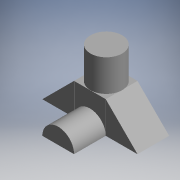
# Autodesk Inventor part: orthographic1
Saved by Autodesk Inventor 2017 (Build 210142000, 142)
## iProperties
Part Number: orthographic1
Material: Generic
Document SubType Name: Modeling
Designer: qthuynh
Appearance: Generic
Author: qthuynh
Autodesk Inventor part; units mm, degrees
ref_plane "YZ Plane" through (0, 0, 0) normal (1, 0, 0) x (0, 1, 0)
ref_plane "XZ Plane" through (0, 0, 0) normal (0, 1, 0) x (-1, 0, 0)
sketch "Sketch1" plane through (0, 0, 0) normal (0, 0, 1) x (1, 0, 0)
  line L0 (0, 0) -> (25.4, 0)
  line L1 (25.4, 0) -> (25.4, 25.4)
  line L2 (25.4, 25.4) -> (0, 25.4)
  line L3 (0, 25.4) -> (0, 0)
  line L4 (25.4, 0) -> (50.8, 0)
  line L5 (50.8, 0) -> (25.4, 25.4)
  line L6 (0, 0) -> (-25.4, 0)
  line L7 (-25.4, 0) -> (0, 25.4)
  dimension "d0" = 25.4
  dimension "d1" = 25.4
  dimension "d2" = 25.4
  dimension "d3" = 25.4
  constraints: 16 end point, 2 horizontal, 2 parallel, 2 perpendicular, 2 point on line
  measures "d0" distance of L2.end L1.end
  measures "d1" distance of L1.end L0.end
  measures "d2" distance of L0.end L4.end
  measures "d3" distance of L0.start L6.end
extrude "Extrusion1" add sketch "Sketch1" along normal blind 25.4 contours L3 L2 L1 L0
chamfer "Chamfer1" distance 0.3 angle 45 2 edges at (25.4, 12.7, 25.4) (0, 12.7, 25.4)
sketch "Sketch2" plane through (0, 0, 25.4) normal (0, 0, 1) x (1, 0, 0)
  line L0 (0, 0) -> (-25.4, 0)
  line L1 (0, 25.4) -> (0, 0) projected
  line L2 (-25.4, 0) -> (0, 25.4)
  line L3 (25.4, 0) -> (50.8, 0)
  line L4 (50.8, 0) -> (25.4, 25.4)
  dimension "d9" = 25.4
  dimension "d10" = 25.4
  constraints: 8 end point, 2 horizontal
  measures "d9" distance of L0.start L0.end
  measures "d10" distance of L3.start L3.end
extrude "Extrusion2" add sketch "Sketch2" against normal blind 25.4
sketch "Sketch3" plane through (0, 0, 25.4) normal (0, 0, 1) x (1, 0, 0)
  line L0 (-25.4, 0) -> (25.4, 0) projected
  line L1 (25.4, 0) -> (50.8, 0)
  line L2 (25.4, 0) -> (25.4, 25.4) projected
  line L3 (50.8, 0) -> (25.4, 25.4)
  point P0 (0, 0)
  dimension "d13" = 25.4
  constraints: 4 end point, 1 horizontal
  measures "d13" distance of L0.end L1.end
extrude "Extrusion3" add sketch "Sketch3" against normal blind 25.4
sketch "Sketch4" plane through (0, 0, 25.4) normal (0, 0, 1) x (1, 0, 0)
  line L0 (0.3, 0) -> (25.1, 0) projected
  circle A0 centre (12.7, 0) radius 12.7
  point P0 (0, 0)
  dimension "d16" = 25.4
  constraints: 1 centre point, 1 midpoint
  measures "d16" diameter of A0
extrude "Extrusion4" add sketch "Sketch4" along normal blind 25.4
ref_plane "Work Plane1" through (0, 0, 25.4) normal (0, 0, 1) x (1, 0, 0)
sketch "Sketch5" plane through (0, 0, 25.4) normal (0, 0, 1) x (1, 0, 0)
  line L0 (0, 0) -> (-25.4, 0) projected
  line L1 (0, 0) -> (42.4435, 0)
  line L2 (42.4435, 0) -> (42.4435, -16.3705)
  line L3 (42.4435, -16.3705) -> (0, -16.3705)
  line L4 (0, -16.3705) -> (0, 0)
  circle A0 centre (12.7, 0) radius 12.7 projected
  constraints: 8 end point, 2 perpendicular, 1 horizontal, 1 horizontal alignment, 1 vertical
extrude "Extrusion5" cut sketch "Sketch5" along normal blind 25.4 contours A0 L1 L2 L3 L4 | L1 A0 picked at (10.2952, -3.484)
sketch "Sketch6" plane through (0.3, 25.4, 25.4) normal (0, 1, 0) x (1, 0, 0)
  point P0 (-0.3, 25.4)
sketch "Sketch7" plane through (0.3, 25.4, 25.4) normal (0, 1, 0) x (1, 0, 0)
  point P0 (-0.3, 25.4)
sketch "Sketch8" plane through (0.3, 25.4, 25.4) normal (0, 1, 0) x (1, 0, 0)
  circle A0 centre (12.7153, 12.8448) radius 12.7
  point P0 (-0.3, 25.4)
  dimension "d22" = 25.4
  constraints: 1 centre point
  measures "d22" diameter of A0
extrude "Extrusion6" add sketch "Sketch8" along normal blind 25.4
body "Solid1"
